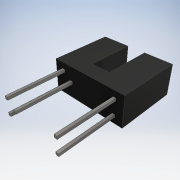
# Autodesk Inventor part: GP1A52HRJ00F (Large slot detector)
Saved by Autodesk Inventor 2018 (Build 220112000, 112)
## iProperties
Created: 2018-01-29
Part Number: GP1A52HRJ00F (Large slot detector)
Material: Generic
Document SubType Name: Modeling
Designer: Moochster
Density: 1 g/cm^3
Appearance: Glossy - Black
Author: Moochster
Autodesk Inventor part; units mm, degrees
ref_plane "YZ Plane" through (0, 0, 0) normal (1, 0, 0) x (0, 1, 0)
ref_plane "XZ Plane" through (0, 0, 0) normal (0, 1, 0) x (-1, 0, 0)
ref_plane "XY Plane" through (0, 0, 0) normal (0, 0, 1) x (1, 0, 0)
sketch "Sketch1" plane through (0, 0, 0) normal (0, 0, 1) x (1, 0, 0)
  line L0 (0, 0) -> (0, 10)
  line L1 (0, 10) -> (4.6, 10)
  line L2 (4.6, 10) -> (4.6, 2.5)
  line L3 (4.6, 2.5) -> (7.6, 2.5)
  line L4 (7.6, 2.5) -> (7.6, 10)
  line L5 (7.6, 10) -> (12.2, 10)
  line L6 (12.2, 10) -> (12.2, 0)
  line L7 (12.2, 0) -> (0, 0)
  dimension "d0" = 12.2
  dimension "d1" = 10
  dimension "d2" = 7.5
  dimension "d3" = 3
  constraints: 16 end point, 6 perpendicular, 2 point on line, 1 collinear, 1 vertical
  measures "d0" distance of L6.end L0.start
  measures "d1" distance of L0.start L0.end
  measures "d2" distance of L1.end L2.end
  measures "d3" distance of L2.end L3.end
extrude "Extrusion1" add sketch "Sketch1" along normal blind 5
sketch "Sketch2" plane through (0, 0, 0) normal (0, -1, 0) x (1, 0, 0)
  line L0 (0, 0) -> (0, 5) projected
  line L1 (1.5, 3.77) -> (10.7, 3.77) construction
  line L2 (0, 5) -> (12.2, 5) construction
  line L3 (1.275, 3.995) -> (1.725, 3.995)
  line L4 (1.725, 3.995) -> (1.725, 3.545)
  line L5 (1.725, 3.545) -> (1.275, 3.545)
  line L6 (1.275, 3.545) -> (1.275, 3.995)
  line L7 (1.275, 3.995) -> (1.725, 3.545) construction
  line L8 (1.725, 3.995) -> (1.275, 3.545) construction
  point P0 (1.5, 1.23)
  point P1 (3, 2.5)
  point P2 (10.7, 1.23)
  point P3 (0, 2.5)
  point P4 (6.1, 3.77)
  point P5 (6.1, 5)
  dimension "d6" = 1.27
  dimension "d7" = 1.27
  dimension "d8" = 1.5
  dimension "d9" = 9.2
  dimension "d10" = 0.45
  dimension "d11" = 0.45
  constraints: 14 end point, 5 midpoint, 3 horizontal alignment, 3 vertical alignment, 2 horizontal, 2 parallel, 1 perpendicular
  measures "d6" vertical distance of point (3, 2.5) L1.start
  measures "d7" vertical distance of point (3, 2.5) point (1.5, 1.23)
  measures "d8" horizontal distance of L1.start point (3, 2.5)
  measures "d9" distance of L1.end L1.start
  measures "d10" distance of L3.start L3.end
  measures "d11" distance of L5.end L3.start
extrude "Extrusion2" add sketch "Sketch2" along normal blind 9
pattern_sketch "Sketch Driven Pattern1" of "Extrusion2" from (1.5, 0, 3.77) copies at (1.5, 0, 1.23) at (3, 0, 2.5) at (10.7, 0, 3.77) at (10.7, 0, 1.23)
body "Solid1"
